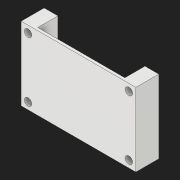
# Autodesk Inventor part: BP010
Saved by Autodesk Inventor 2017 SP1 (Build 210196100, 196)
## iProperties
Created: 2018-03-11
Part Number: BP010
Material: ABS Plastic
Document SubType Name: Modeling
Designer: Zach
Density: 1.06 g/cm^3
Appearance: CR White
Author: Zach
Autodesk Inventor part; units mm, degrees
ref_plane "YZ Plane" through (0, 0, 0) normal (1, 0, 0) x (0, 1, 0)
ref_plane "XZ Plane" through (0, 0, 0) normal (0, 1, 0) x (-1, 0, 0)
ref_plane "XY Plane" through (0, 0, 0) normal (0, 0, 1) x (1, 0, 0)
sketch "Sketch1" plane through (0, 0, 0) normal (0, 0, 1) x (1, 0, 0)
  line L0 (0, 0) -> (110, 0) construction
  line L1 (110, 0) -> (110, 65) construction
  line L2 (110, 65) -> (0, 65) construction
  line L3 (0, 65) -> (0, 0) construction
  circle A0 centre (0, 65) radius 1.5
  circle A1 centre (0, 0) radius 1.5
  circle A2 centre (110, 0) radius 1.5
  circle A3 centre (110, 65) radius 1.5
  line L4 (-7.5, 72.5) -> (7.5, 72.5)
  line L5 (7.5, 72.5) -> (7.5, -7.5)
  line L6 (7.5, -7.5) -> (-7.5, -7.5)
  line L7 (-7.5, -7.5) -> (-7.5, 72.5)
  line L8 (102.5, 72.5) -> (117.5, 72.5)
  line L9 (117.5, 72.5) -> (117.5, -7.5)
  line L10 (117.5, -7.5) -> (102.5, -7.5)
  line L11 (102.5, -7.5) -> (102.5, 72.5)
  point P0 (7.5, 32.5)
  point P1 (0, 32.5)
  point P2 (102.5, 32.5)
  point P3 (110, 32.5)
  point P4 (0, 72.5)
  point P5 (110, 72.5)
  dimension "d0" = 110
  dimension "d1" = 65
  dimension "d2" = 3
  dimension "d3" = 3
  dimension "d4" = 3
  dimension "d5" = 3
  dimension "d6" = 15
  dimension "d7" = 15
  dimension "d8" = 80
  constraints: 24 end point, 6 midpoint, 6 parallel, 4 centre point, 4 coincident, 3 horizontal, 3 horizontal alignment, 3 perpendicular, 2 vertical alignment
  measures "d0" distance of L2.end L1.end
  measures "d1" distance of L1.end L0.end
  measures "d2" diameter of A0
  measures "d3" diameter of A1
  measures "d4" diameter of A2
  measures "d5" diameter of A3
  measures "d6" distance of L4.start L4.end
  measures "d7" distance of L8.start L8.end
  measures "d8" distance of L6.end L4.start
extrude "Extrusion1" add sketch "Sketch1" along normal blind 22
sketch "Sketch2" plane through (0, 0, 22) normal (0, 0, 1) x (1, 0, 0)
  circle A0 centre (0, 65) radius 1.5 projected
  circle A1 centre (0, 0) radius 1.5 projected
  circle A2 centre (110, 0) radius 1.5 projected
  circle A3 centre (110, 65) radius 1.5 projected
  line L0 (-7.5, 72.5) -> (-7.5, -7.5) projected
  line L1 (7.5, 72.5) -> (-7.5, 72.5) projected
  line L2 (102.5, -7.5) -> (117.5, -7.5) projected
  line L3 (117.5, -7.5) -> (117.5, 72.5) projected
  line L4 (-7.5, 72.5) -> (117.5, 72.5)
  line L5 (117.5, 72.5) -> (117.5, -7.5)
  line L6 (117.5, -7.5) -> (-7.5, -7.5)
  line L7 (-7.5, -7.5) -> (-7.5, 72.5)
  constraints: 8 end point, 2 parallel, 1 horizontal, 1 perpendicular
extrude "Extrusion2" add sketch "Sketch2" along normal blind 3
sketch "Sketch3" plane through (0, 0, 25) normal (0, 0, 1) x (1, 0, 0)
  circle A0 centre (0, 65) radius 1.5 projected
  circle A1 centre (110, 65) radius 1.5 projected
  circle A2 centre (110, 0) radius 1.5 projected
  circle A3 centre (0, 0) radius 1.5 projected
  circle A4 centre (0, 65) radius 1.5 projected
  circle A5 centre (0, 65) radius 4
  circle A6 centre (0, 0) radius 1.5 projected
  circle A7 centre (0, 0) radius 4
  circle A8 centre (110, 0) radius 1.5 projected
  circle A9 centre (110, 0) radius 4
  circle A10 centre (110, 65) radius 4
  dimension "d13" = 8
  dimension "d14" = 8
  dimension "d15" = 8
  dimension "d16" = 8
  constraints: 4 centre point, 4 coincident
  measures "d13" diameter of A5
  measures "d14" diameter of A7
  measures "d15" diameter of A9
  measures "d16" diameter of A10
extrude "Extrusion3" cut sketch "Sketch3" against normal blind 20 contours A0 | A1 | A2 | A3 | A5 | A7 | A9 | A10
body "Solid1"
